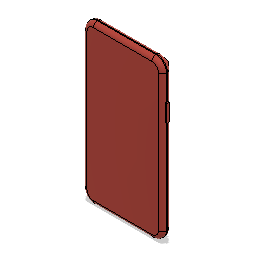
IPHONE_11 (PENDING CHECK) v10 (Autodesk Fusion 360 design; units mm, degrees)
Autodesk Fusion 360 part; units mm, degrees
sketch "Sketch1" plane through (0, 0, 0) normal (0, 0, 1) x (1, 0, 0)
  line L0 (37.85, 75.45) -> (-37.85, 75.45)
  line L1 (-37.85, 75.45) -> (-37.85, -75.45)
  line L2 (-37.85, -75.45) -> (37.85, -75.45)
  line L3 (37.85, -75.45) -> (37.85, 75.45)
  line L4 (37.85, 75.45) -> (-37.85, -75.45) construction
  line L5 (-37.85, 75.45) -> (37.85, -75.45) construction
  dimension "d1" = 75.7
  dimension "d2" = 150.9
  constraint horizontal L0
  constraint perpendicular L0 L1
  constraint parallel L0 L2
  constraint parallel L1 L3
  constraint coincident L4 origin
  constraint coincident L5 origin
  measures "d1" distance of L1.end L2.end
  measures "d2" distance of L0.end L1.end
extrude "Extrude1" add sketch "Sketch1" along normal blind 8.3 makes body 1
sketch "Sketch3" plane through (0, 0, 0) normal (0, 0, -1) x (1, 0, 0)
  line L0 (6.85, -39.45) -> (33.85, -39.45)
  line L1 (33.85, -39.45) -> (33.85, -70.45)
  line L2 (33.85, -70.45) -> (6.85, -70.45)
  line L3 (6.85, -70.45) -> (6.85, -39.45)
  line L4 (6.85, -39.45) -> (33.85, -70.45) construction
  line L5 (33.85, -39.45) -> (6.85, -70.45) construction
  line L6 (-37.85, 75.45) -> (-37.85, -75.45)
  line L7 (-37.85, -75.45) -> (37.85, -75.45)
  line L8 (37.85, -75.45) -> (37.85, 75.45)
  line L9 (37.85, 75.45) -> (-37.85, 75.45)
  point P0 (20.35, -54.95)
  dimension "d9" = 27
  dimension "d10" = 31
  dimension "d31" = 5
  dimension "d32" = 4
  constraint horizontal L0
  constraint perpendicular L0 L1
  constraint parallel L0 L2
  constraint parallel L1 L3
  constraint coincident L4 P0
  constraint coincident L5 P0
  measures "d9" distance of L0.start L0.end
  measures "d10" distance of L0.start L2.end
  measures "d31" distance of L2 L7
  measures "d32" distance of L1 L8
extrude "Extrude2" add sketch "Sketch3" along normal blind 1.5 contours L0 L1 L2 L3 bodies 1
fillet "Fillet2" radius 3 4 edges at (33.85, 70.45, -0.75) (33.85, 39.45, -0.75) (6.85, 70.45, -0.75) (6.85, 39.45, -0.75) on bodies 1
sketch "Sketch4" plane through (37.85, 0, 0) normal (1, 0, 0) x (0, 0, -1)
  line L0 (0, -75.45) -> (0, 75.45)
  line L1 (-8.3, 75.45) -> (-8.3, -75.45)
  line L2 (1.5, 42.45) -> (1.5, 39.45)
  line L3 (1.5, 39.45) -> (0, 39.45)
  line L4 (1.5, 42.45) -> (1.5, 67.45)
  line L5 (1.5, 70.45) -> (1.5, 67.45)
  line L6 (0, 70.45) -> (1.5, 70.45)
  line L7 (0, 75.45) -> (0, 70.45)
  line L8 (-8.3, 75.45) -> (-8.3, -75.45)
  line L9 (-4.15, 75.45) -> (-4.15, -75.45) construction
  line L10 (-2.9, 24.2) -> (-5.4, 24.2)
  line L11 (-5.4, 24.2) -> (-5.4, 40.7)
  line L12 (-5.4, 40.7) -> (-2.9, 40.7)
  line L13 (-2.9, 40.7) -> (-2.9, 24.2)
  line L14 (-2.9, 24.2) -> (-5.4, 40.7) construction
  line L15 (-5.4, 24.2) -> (-2.9, 40.7) construction
  line L16 (0, 75.45) -> (-8.3, 75.45)
  line L17 (-8.3, -75.45) -> (0, -75.45)
  line L18 (0, -75.45) -> (-8.3, -75.45)
  line L19 (0, 75.45) -> (-8.3, 75.45)
  line L20 (0, 39.45) -> (0, -75.45)
  point P0 (-4.15, 32.45)
  dimension "d20" = 2.5
  dimension "d21" = 16.5
  dimension "d33" = 34.75
  constraint horizontal L10
  constraint perpendicular L10 L11
  constraint parallel L10 L12
  constraint parallel L11 L13
  constraint coincident L14 P0
  constraint coincident L15 P0
  constraint coincident L9 P0
  constraint midpoint L9.end L17
  constraint perpendicular L9 L17
  constraint midpoint L9.start L19
  measures "d20" distance of L10.start L10.end
  measures "d21" distance of L10.start L12.end
  measures "d33" distance of L12 L19
extrude "Extrude3" add sketch "Sketch4" along normal blind 1 contours L10 L11 L12 L13 bodies 1
sketch "Sketch5" plane through (-37.85, 0, 0) normal (-1, 0, 0) x (0, 0, 1)
  line L0 (8.3, -75.45) -> (8.3, 75.45)
  line L1 (0, 75.45) -> (0, -75.45)
  line L2 (-1.5, 67.45) -> (-1.5, 70.45)
  line L3 (-1.5, 67.45) -> (-1.5, 42.45)
  line L4 (-1.5, 39.45) -> (-1.5, 42.45)
  line L5 (0, 39.45) -> (-1.5, 39.45)
  line L6 (-1.5, 70.45) -> (0, 70.45)
  line L7 (0, -75.45) -> (0, 39.45)
  line L8 (8.3, -75.45) -> (8.3, 75.45)
  line L9 (4.15, 75.45) -> (4.15, -75.45) construction
  line L10 (5.35, 34.25) -> (2.95, 34.25)
  line L11 (2.95, 34.25) -> (2.95, 44.75)
  line L12 (2.95, 44.75) -> (5.35, 44.75)
  line L13 (5.35, 44.75) -> (5.35, 34.25)
  line L14 (5.35, 34.25) -> (2.95, 44.75) construction
  line L15 (2.95, 34.25) -> (5.35, 44.75) construction
  line L16 (0, 32.75) -> (8.3, 32.75) construction
  line L17 (2.95, 31.25) -> (2.95, 20.75)
  line L18 (2.95, 20.75) -> (5.35, 20.75)
  line L19 (5.35, 31.25) -> (2.95, 31.25)
  line L20 (5.35, 20.75) -> (5.35, 31.25)
  line L21 (0, -75.45) -> (8.3, -75.45)
  line L22 (8.3, 75.45) -> (0, 75.45)
  line L23 (0, -75.45) -> (8.3, -75.45)
  line L24 (0, 75.45) -> (8.3, 75.45)
  line L25 (0, 70.45) -> (0, 75.45)
  point P0 (4.15, 39.5)
  dimension "d25" = 1.5
  dimension "d26" = 10.5
  dimension "d27" = 2.4
  dimension "d38" = 30.7
  constraint horizontal L10
  constraint perpendicular L10 L11
  constraint parallel L10 L12
  constraint parallel L11 L13
  constraint coincident L14 P0
  constraint coincident L15 P0
  constraint coincident L9 P0
  constraint coincident L7 L16.start
  constraint coincident L8 L16.end
  constraint perpendicular L8 L16
  constraint symmetric L10.start L16 L19.start
  constraint symmetric L10.end L16 L17.start
  constraint symmetric L11.end L16 L17.end
  constraint symmetric L12.end L16 L18.end
  constraint midpoint L9.start L22
  constraint perpendicular L9 L22
  constraint midpoint L9.end L23
  measures "d25" distance of L10 L16
  measures "d26" distance of L10.start L12.end
  measures "d27" distance of L10.start L10.end
  measures "d38" distance of L12 L22
extrude "Extrude4" add sketch "Sketch5" along normal blind 1 contours L10 L11 L12 L13 | L17 L18 L19 L20 bodies 1
fillet "Fillet1" radius 10 4 edges at (-37.85, 75.45, 4.15) (37.85, 75.45, 4.15) (37.85, -75.45, 4.15) (-37.85, -75.45, 4.15) on bodies 1
fillet "Fillet4" radius 3.75 16 edges at (-34.9211, 72.5211, 0) (-37.85, 0, 0) (-34.9211, -72.5211, 0) (0, -75.45, 0) (34.9211, -72.5211, 0) (37.85, 0, 0) (34.9211, 72.5211, 0) (0, 75.45, 0) (37.85, 0, 8.3) (34.9211, 72.5211, 8.3) (0, 75.45, 8.3) (-34.9211, 72.5211, 8.3) (-37.85, 0, 8.3) (-34.9211, -72.5211, 8.3) (0, -75.45, 8.3) (34.9211, -72.5211, 8.3) on bodies 1
copy_body "CopyPasteBodies1" bodies 1 makes body 2
move_body "Move1" bodies 2 to x (1, 0, 0) y (0, 1, 0) z (0, 0, 1) at (0, 0, 0)
scale "Scale1" factors (1.006, 1.003, 1.051) about (9.85, 39.45, 0) bodies 2
copy_body "CopyPasteBodies2" bodies 2 makes body 3
move_body "Move2" bodies 3 to x (-1, 0, 0) y (0, -1, 0) z (0, 0, 1) at (0.0744, -0.228, 0)
hidden bodies 1 3
equation "d25 = ( 3 / 2 ) * 1 mm"
named bodies: "IPHONE_11", "IPHONE_14P", "IPHONE_11_FIT", "IPHONE_14P_FIT", "IPHONE_11_FIT REVERSED"
